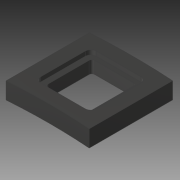
# Autodesk Inventor part: led_ring_assembly_jig
Saved by Autodesk Inventor 2019 (Build 230136000, 136)
## iProperties
Created: 2019-02-28
Part Number: led_ring_assembly_jig
Material: ABS Plastic
Document SubType Name: Modeling
Designer: WW
Density: 1.06 g/cm^3
Appearance: Smooth - Black
Author: WW
Autodesk Inventor part; units mm, degrees
ref_plane "YZ Plane" through (0, 0, 0) normal (1, 0, 0) x (0, 1, 0)
ref_plane "XZ Plane" through (0, 0, 0) normal (0, 1, 0) x (-1, 0, 0)
ref_plane "XY Plane" through (0, 0, 0) normal (0, 0, 1) x (1, 0, 0)
sketch "Sketch1" plane through (0, 0, 0) normal (0, 1, 0) x (-1, 0, 0)
  circle A0 centre (0, 0) radius 102.5
  circle A1 centre (0, 0) radius 117.5
  circle A2 centre (0, 0) radius 110 construction
  dimension "d0" = 15
  dimension "nomdia" = 220
  dimension "d19" = 7.5
  constraints: 3 centre point, 3 coincident
  measures "d0" radial gap between concentric circles of A0 A1
  measures "nomdia" diameter of A2
  measures "d19" radial gap between concentric circles of A1 A2
extrude "Extrusion1" add sketch "Sketch1" along normal blind 3
sketch "Sketch2" plane through (0, 3, 0) normal (0, 1, 0) x (1, 0, 0)
  circle A0 centre (0, 0) radius 102.5 construction
  circle A1 centre (0, 0) radius 117.5 construction
  line L0 (0, 117.5) -> (0, 102.5) construction
  line L1 (-5, 105) -> (5, 105)
  line L2 (5, 105) -> (5, 115)
  line L3 (5, 115) -> (-5, 115)
  line L4 (-5, 115) -> (-5, 105)
  line L5 (-5, 105) -> (5, 115) construction
  line L6 (5, 105) -> (-5, 115) construction
  point P0 (0, 110)
  point P1 (0, 110)
  dimension "d5" = 10
  dimension "d6" = 10
  constraints: 14 end point, 3 midpoint, 3 vertical alignment, 2 parallel, 1 horizontal, 1 perpendicular, 1 vertical, 2 other
  measures "d5" distance of L3.end L2.end
  measures "d6" distance of L2.end L1.end
extrude "Extrusion2" cut sketch "Sketch2" against normal blind 0.8
fillet "Fillet1" radius 1 4 edges at (5, 2.6, -115) (5, 2.6, -105) (-5, 2.6, -115) (-5, 2.6, -105)
sketch "Sketch3" plane through (0, 2.2, 0) normal (0, 1, 0) x (1, 0, 0)
  arc A0 (-5, 106) -> (-4, 105) centre (-4, 106) ccw construction
  line L0 (4, 105) -> (-4, 105) construction
  arc A1 (4, 105) -> (5, 106) centre (4, 106) ccw construction
  line L1 (5, 114) -> (5, 106) construction
  arc A2 (5, 114) -> (4, 115) centre (4, 114) ccw construction
  line L2 (-4, 115) -> (4, 115) construction
  arc A3 (-4, 115) -> (-5, 114) centre (-4, 114) ccw construction
  line L3 (-5, 106) -> (-5, 114) construction
  line L4 (-4, 105) -> (4, 105)
  line L5 (4, 105) -> (4, 115)
  line L6 (4, 115) -> (-4, 115)
  line L7 (-4, 115) -> (-4, 105)
  line L8 (-4, 105) -> (4, 115) construction
  line L9 (4, 105) -> (-4, 115) construction
  line L10 (-4, 115) -> (4, 115) construction
  line L11 (-4, 105.8) -> (4, 105.8)
  line L12 (4, 105.8) -> (4, 114.2)
  line L13 (4, 114.2) -> (-4, 114.2)
  line L14 (-4, 114.2) -> (-4, 105.8)
  line L15 (-4, 105.8) -> (4, 114.2) construction
  line L16 (4, 105.8) -> (-4, 114.2) construction
  line L17 (4, 105) -> (-4, 105) construction
  point P0 (0, 0)
  point P1 (0, 110)
  point P2 (0, 115)
  point P3 (0, 110)
  dimension "d10" = 8
  dimension "d13" = 0.8
  constraints: 24 end point, 6 midpoint, 4 parallel, 3 point on line, 2 horizontal, 2 perpendicular, 1 vertical alignment
  measures "d10" distance between parallel lines of L5 L7
  measures "d13" distance between parallel lines of L6 L13
extrude "Extrusion3" cut sketch "Sketch3" along normal through all both and the other way through all contours L7 L13 L5 L11
fillet "Fillet2" radius 0.5 4 edges at (-4, 1.1, -114.2) (4, 1.1, -114.2) (4, 1.1, -105.8) (-4, 1.1, -105.8)
pattern_circular "Circular Pattern1" count 40 over 360 about axis through (0, 0, 0) along (0, 1, 0) of "Extrusion3", "Extrusion2", "Fillet1", "Fillet2"
sketch "Sketch4" plane through (0, 3, 0) normal (0, 1, 0) x (1, 0, 0)
  line L0 (-4, 106.3) -> (-4, 113.7) construction
  arc A0 (-3.5, 114.2) -> (-4, 113.7) centre (-3.5, 113.7) ccw construction
  line L1 (-3.5, 114.2) -> (3.5, 114.2) construction
  arc A1 (4, 113.7) -> (3.5, 114.2) centre (3.5, 113.7) ccw construction
  line L2 (4, 113.7) -> (4, 106.3) construction
  arc A2 (3.5, 105.8) -> (4, 106.3) centre (3.5, 106.3) ccw construction
  line L3 (3.5, 105.8) -> (-3.5, 105.8) construction
  arc A3 (-4, 106.3) -> (-3.5, 105.8) centre (-3.5, 106.3) ccw construction
  arc A4 (-5, 106) -> (-4, 105) centre (-4, 106) ccw construction
  line L4 (4, 105) -> (-4, 105) construction
  arc A5 (4, 105) -> (5, 106) centre (4, 106) ccw construction
  line L5 (5, 114) -> (5, 106) construction
  arc A6 (5, 114) -> (4, 115) centre (4, 114) ccw construction
  line L6 (-4, 115) -> (4, 115) construction
  arc A7 (-4, 115) -> (-5, 114) centre (-4, 114) ccw construction
  line L7 (-5, 106) -> (-5, 114) construction
  line L8 (-7.5, 101.522) -> (7.5, 101.522)
  line L9 (7.5, 101.522) -> (7.5, 118.478)
  line L10 (7.5, 118.478) -> (-7.5, 118.478)
  line L11 (-7.5, 118.478) -> (-7.5, 101.522)
  line L12 (-7.5, 101.522) -> (7.5, 118.478) construction
  line L13 (7.5, 101.522) -> (-7.5, 118.478) construction
  circle A8 centre (0, 0) radius 190.5451
  point P0 (0, 110)
  dimension "d20" = 15
  constraints: 12 end point, 2 midpoint, 2 parallel, 1 centre point, 1 coincident, 1 horizontal, 1 perpendicular
  measures "d20" distance of L10.end L9.end
extrude "Extrusion4" cut sketch "Sketch4" against normal through all
body "Solid1"
